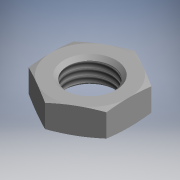
# Autodesk Inventor part: SLZ_63_Mutter_M16#
Saved by Autodesk Inventor 2017.3 (Build 213256000, 256)
## iProperties
Part Number: SLZ_63_Mutter_M16#
Material: Generic
Catalog Web Link: www.cadenas.de
Description: Mutter_SLZ63-Control-Tec
Vendor: ROSEKRIEGER
Document SubType Name: Modeling
Designer: partserver
Manufacturer: ROSEKRIEGER
Mass: 2.72048 g
Surface Area: 16.3265 cm^2
Volume: 2.72048 cm^3
Density: 1 g/cm^3
Appearance: PSOLRGB-191-191-191
Category: PARTsolutions
Company: ROSEKRIEGER
Title: SLZ_63_Mutter_M16#
Author: Cadenas PARTsolutions
Comments: Control-Tec
PSOL_IDENT_0: {$CADENAS_DATA\23d-libs\rose_krieger\linearkomponenten\pool_lineartechnik\_hubsaeule_zyliinder\elekt
PSOL_IDENT_1: rozylinder\elekzyl_slz63\parts\slz63_plfl_mutter_16.prj},182 {VTYP=3D},{NB=SLZ_63_Mutter_M16#},{LINA=
PSOL_IDENT_2: SLZ_63_Mutter_M16#},{NN=Mutter_SLZ63},{DATE=02.12.2020 11:16:25},{GEOMDATE=22.06.2016 13:05:45},{VER
PSOL_IDENT_3: SION=},{LINEID=10},{WBVAR=},{WBNUMERIC=}  {NB=SLZ_63_Mutter_M16#},{LINA=SLZ_63_Mutter_M16#},{KT=DUMM
PSOL_IDENT_4: Y},{IDNR=},{CODE=TQ3},{ARTIKEL=Elektrozylinder },{TYPE=SLZ 63 KG P PL},{BEST=SLZ_63_Mutter_M16},{VAR
PSOL_IDENT_5: IANTE=PL},{SPINDEL=KG 25x10},{SPINDELCODE=3.000},{SCHUTZARTVIS=IP54},{SCHUTZART=1},{HUB1=0,[0:100]},
PSOL_IDENT_6: {HINWEINBAUX=Hub + 288,5 mm},{DUMMYDURCH=10.000},{DUMMYLAENG=20.000},{HILFEHUB=105},{LAENDOPPROFIL=1
PSOL_IDENT_7: 84.500},{RF=1.000},{GRUNDKOE=288.500},{A=100},{B=80},{C=100},{D=125},{E=238},{F=40},{G=M16x1.5},{H=1
PSOL_IDENT_8: 04},{K=125},{L=105},{M=48},{N=56.5},{O=86},{P=18.5},{PPATH=sbl_lz70p_plfl.prj}
NB: SLZ_63_Mutter_M16#
NN: Mutter_SLZ63
NT: Control-Tec
NBSYN: $BEST.#
LINA: SLZ_63_Mutter_M16#
CATALOG: RK Rose+Krieger
ARTIKEL: Elektrozylinder
TYPE: SLZ 63 KG P PL
BEST: SLZ_63_Mutter_M16
VARIANTE: PL
SPINDEL: KG 25x10
SPINDELCODE: 3
SCHUTZARTVIS: IP54
SCHUTZART: 1
HUB1: 0,[0:100]
HINWEINBAUX: Hub + 288,5 mm
DUMMYDURCH: 10
DUMMYLAENG: 20
HILFEHUB: 105
LAENDOPPROFIL: 184.5
GRUNDKOE: 288.5
A: 100
B: 80
C: 100
D: 125
E: 238
F: 40
G: M16x1.5
H: 104
K: 125
L: 105
M: 48
N: 56.5
O: 86
P: 18.5
SUPPLIER: ROSEKRIEGER
ARTICLENO: SLZ_63_Mutter_M16#
BOMINFO: SLZ_63_Mutter_M16#
CREATOR: CADENAS GmbH
Autodesk Inventor part; units mm, degrees
sketch "Sketch_3" plane through (0, 0, 0) normal (1, 0, 0) x (0, 0, -1)
  line L0 (0, 0) -> (-8, 0)
  line L1 (-8, 0) -> (-8, 12)
  line L2 (-8, 12) -> (-7.3569, 14.4)
  line L3 (-7.3569, 14.4) -> (-0.6431, 14.4)
  line L4 (-0.6431, 14.4) -> (0, 12)
  line L5 (0, 12) -> (0, 0)
  line L6 (0, 0) -> (-8, 0)
  constraints: 14 end point
revolve "Revolution1" add sketch "Sketch_3" angle 360 about axis through (0, 0, 0) along (0, 0, -1)
sketch "Sketch_2" plane through (0, 0, 0) normal (1, 0, 0) x (0, 0, -1)
  line L0 (0, 0) -> (-8, 0)
  line L1 (-8, 0) -> (-8, 8)
  line L2 (-8, 8) -> (-6.9175, 6.9175)
  line L3 (-6.9175, 6.9175) -> (-1.0825, 6.9175)
  line L4 (-1.0825, 6.9175) -> (0, 8)
  line L5 (0, 8) -> (0, 0)
  line L6 (0, 0) -> (-8, 0)
  constraints: 14 end point
revolve "Revolution2" cut sketch "Sketch_2" angle 360 about axis through (0, 0, 0) along (0, 0, -1)
thread "Thread1" size "M16x2" class "6H" standard "ISO Metric profile" full length
sketch "Sketch_1" plane through (0, 0, 0) normal (0, 0, 1) x (1, 0, 0)
  line L0 (-24, -24) -> (24, -24)
  line L1 (24, -24) -> (24, 24)
  line L2 (24, 24) -> (-24, 24)
  line L3 (-24, 24) -> (-24, -24)
  line L4 (-12, -6.9282) -> (0, -13.8564)
  line L5 (0, -13.8564) -> (12, -6.9282)
  line L6 (12, -6.9282) -> (12, 6.9282)
  line L7 (12, 6.9282) -> (0, 13.8564)
  line L8 (0, 13.8564) -> (-12, 6.9282)
  line L9 (-12, 6.9282) -> (-12, -6.9282)
  constraints: 20 end point
extrude "Extrusion1" cut sketch "Sketch_1" along normal blind 8
ref_plane "MUTTER_XY" through (0, 0, 0) normal (0, 0, 1) x (1, 0, 0)
ref_plane "MUTTER_YZ" through (0, 0, 0) normal (1, 0, 0) x (0, 1, 0)
ref_plane "MUTTER_ZX" through (0, 0, 0) normal (0, 1, 0) x (0, 0, 1)
body "Solid1"
